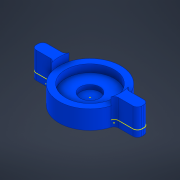
# Autodesk Inventor part: caja_down
Saved by Autodesk Inventor 2021 (Build 250183000, 183)
## iProperties
Created: 2021-12-14
Part Number: caja_down
Material: Generic
Document SubType Name: Modeling
Designer: Juan M. Casillas
Density: 1 g/cm^3
Appearance: Default
Author: Juan M. Casillas
Autodesk Inventor part; units mm, degrees
ref_plane "YZ Plane" through (0, 0, 0) normal (1, 0, 0) x (0, 1, 0)
ref_plane "XZ Plane" through (0, 0, 0) normal (0, 1, 0) x (-1, 0, 0)
ref_plane "XY Plane" through (0, 0, 0) normal (0, 0, 1) x (1, 0, 0)
sketch "Sketch2" plane through (0, 0, 0) normal (0, 1, 0) x (-1, 0, 0)
  circle A0 centre (0, 0) radius 11.1
  circle A1 centre (0, 0) radius 14.1
  dimension "d5" = 22.2
  dimension "d6" = 3
  constraints: 2 centre point, 1 coincident
  measures "d5" diameter of A0
  measures "d6" radial gap between concentric circles of A0 A1
extrude "Extrusion2" add sketch "Sketch2" along normal blind 3.5
sketch "Sketch3" plane through (0, 0, 0) normal (0, -1, 0) x (1, 0, 0)
  circle A0 centre (0, 0) radius 14.1 projected
  circle A1 centre (0, 0) radius 4.5
  dimension "d9" = 9
  constraints: 1 centre point, 1 coincident
  measures "d9" diameter of A1
extrude "Extrusion3" add sketch "Sketch3" along normal blind 2
sketch "Sketch4" plane through (0, -2, 0) normal (0, -1, 0) x (1, 0, 0)
  line L0 (-22.1, -2.5014) -> (-15.4579, -2.5014)
  line L1 (-15.4587, 2.4986) -> (-22.1, 2.4986)
  line L2 (-24.1, 0.4986) -> (-24.1, -0.5014)
  line L3 (-24.1, -2.5014) -> (-14.1, 2.4986) construction
  line L4 (-14.1, -2.5014) -> (-24.1, 2.4986) construction
  line L5 (-14.1, -2.5014) -> (-13.8763, -2.5014)
  line L6 (-14.1, 2.4986) -> (-13.8769, 2.4986)
  arc A0 (-13.5377, -3.9422) -> (-15.4579, -2.5014) centre (-15.4579, -4.5014) ccw
  arc A1 (-15.4587, 2.4986) -> (-13.5384, 3.9397) centre (-15.4587, 4.4986) ccw
  arc A2 (-24.1, -0.5014) -> (-22.1, -2.5014) centre (-22.1, -0.5014) ccw
  arc A3 (-22.1, 2.4986) -> (-24.1, 0.4986) centre (-22.1, 0.4986) ccw
  line L7 (0, -19.3985) -> (0, 27.2303) construction
  line L8 (22.1, -2.5014) -> (15.4579, -2.5014)
  line L9 (15.4587, 2.4986) -> (22.1, 2.4986)
  line L10 (24.1, 0.4986) -> (24.1, -0.5014)
  arc A4 (15.4579, -2.5014) -> (13.5377, -3.9422) centre (15.4579, -4.5014) ccw
  arc A5 (13.5384, 3.9397) -> (15.4587, 2.4986) centre (15.4587, 4.4986) ccw
  arc A6 (22.1, -2.5014) -> (24.1, -0.5014) centre (22.1, -0.5014) ccw
  arc A7 (24.1, 0.4986) -> (22.1, 2.4986) centre (22.1, 0.4986) ccw
  arc A8 (-13.5377, -3.9422) -> (13.5377, -3.9422) centre (0, 0) ccw
  arc A9 (13.5384, 3.9397) -> (-13.5384, 3.9397) centre (0, 0) ccw
  point P0 (-19.1, -0.0014)
  point P1 (14.1, 0)
  point P2 (-14.1, 0)
  point P3 (-14.1, 0)
  dimension "d13" = 5
  dimension "d14" = 2
  constraints: 22 end point, 20 point on circle, 12 symmetric about line, 10 centre point, 7 point on line, 6 tangent, 3 equal radius, 2 midpoint, 1 parallel, 1 vertical, 4 other
  measures "d13" distance of L3.end L4.start
  measures "d14" radius of A0
extrude "Extrusion4" add sketch "Sketch4" along normal blind 3
sketch "Sketch5" plane through (0, -2, 0) normal (0, 1, 0) x (1, 0, 0)
  arc A0 (-13.5377, 3.9422) -> (-13.5384, -3.9397) centre (0, 0) ccw projected
  arc A1 (-15.4579, 2.5014) -> (-13.5377, 3.9422) centre (-15.4579, 4.5014) ccw projected
  line L0 (-22.1, 2.5014) -> (-15.4579, 2.5014) projected
  arc A2 (-22.1, 2.5014) -> (-24.1, 0.5014) centre (-22.1, 0.5014) ccw projected
  line L1 (-24.1, -0.4986) -> (-24.1, 0.5014) projected
  arc A3 (-24.1, -0.4986) -> (-22.1, -2.4986) centre (-22.1, -0.4986) ccw projected
  line L2 (-15.4587, -2.4986) -> (-22.1, -2.4986) projected
  arc A4 (-13.5384, -3.9397) -> (-15.4587, -2.4986) centre (-15.4587, -4.4986) ccw projected
  arc A5 (13.5384, -3.9397) -> (13.5377, 3.9422) centre (0, 0) ccw projected
  arc A6 (15.4587, -2.4986) -> (13.5384, -3.9397) centre (15.4587, -4.4986) ccw projected
  line L3 (22.1, -2.4986) -> (15.4587, -2.4986) projected
  arc A7 (22.1, -2.4986) -> (24.1, -0.4986) centre (22.1, -0.4986) ccw projected
  line L4 (24.1, 0.5014) -> (24.1, -0.4986) projected
  arc A8 (24.1, 0.5014) -> (22.1, 2.5014) centre (22.1, 0.5014) ccw projected
  line L5 (15.4579, 2.5014) -> (22.1, 2.5014) projected
  arc A9 (13.5377, 3.9422) -> (15.4579, 2.5014) centre (15.4579, 4.5014) ccw projected
extrude "Extrusion5" add sketch "Sketch5" along normal up to surface (5.5 mm away)
sketch "Sketch6" plane through (0, 3.5, 0) normal (0, 1, 0) x (1, 0, 0)
  arc A0 (-15.4579, 2.5014) -> (-13.5377, 3.9422) centre (-15.4579, 4.5014) ccw projected
  line L0 (-22.1, 2.5014) -> (-15.4579, 2.5014) projected
  arc A1 (-22.1, 2.5014) -> (-24.1, 0.5014) centre (-22.1, 0.5014) ccw projected
  line L1 (-24.1, -0.4986) -> (-24.1, 0.5014) projected
  arc A2 (-24.1, -0.4986) -> (-22.1, -2.4986) centre (-22.1, -0.4986) ccw projected
  line L2 (-15.4587, -2.4986) -> (-22.1, -2.4986) projected
  arc A3 (-13.5384, -3.9397) -> (-15.4587, -2.4986) centre (-15.4587, -4.4986) ccw projected
  arc A4 (-13.5377, 3.9422) -> (-13.5384, -3.9397) centre (0, 0) ccw projected
  arc A5 (15.4587, -2.4986) -> (13.5384, -3.9397) centre (15.4587, -4.4986) ccw projected
  line L3 (22.1, -2.4986) -> (15.4587, -2.4986) projected
  arc A6 (22.1, -2.4986) -> (24.1, -0.4986) centre (22.1, -0.4986) ccw projected
  line L4 (24.1, 0.5014) -> (24.1, -0.4986) projected
  arc A7 (24.1, 0.5014) -> (22.1, 2.5014) centre (22.1, 0.5014) ccw projected
  line L5 (15.4579, 2.5014) -> (22.1, 2.5014) projected
  arc A8 (13.5377, 3.9422) -> (15.4579, 2.5014) centre (15.4579, 4.5014) ccw projected
  arc A9 (13.5384, -3.9397) -> (13.5377, 3.9422) centre (0, 0) ccw projected
extrude "Extrusion6" add sketch "Sketch6" along normal blind 3.5
sketch "Sketch1" plane through (0, 0, 0) normal (0, 1, 0) x (-1, 0, 0)
  line L0 (40, 40) -> (-40, 40)
  line L1 (-40, 40) -> (-40, -40)
  line L2 (-40, -40) -> (40, -40)
  line L3 (40, -40) -> (40, 40)
  line L4 (40, 40) -> (-40, -40) construction
  line L5 (-40, 40) -> (40, -40) construction
  point P0 (0, 0)
  dimension "d0" = 80
  dimension "d1" = 80
  constraints: 12 end point, 2 midpoint, 2 parallel, 1 horizontal, 1 perpendicular
  measures "d0" distance of L2.end L1.end
  measures "d1" distance of L1.end L0.end
body "Solid1"
body "Solid2"
